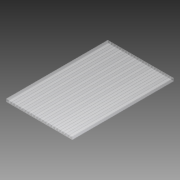
# Autodesk Inventor part: 8 ball polycarb side
Saved by Autodesk Inventor 2012 (Build 160160000, 160)
## iProperties
Created: 2013-10-11
Part Number: 8 ball polycarb side
Material: Default
Document SubType Name: Modeling
Designer: Bryce
Density: 1 g/cm^3
Author: Bryce
Autodesk Inventor part; units mm, degrees
ref_plane "YZ Plane" through (0, 0, 0) normal (1, 0, 0) x (0, 1, 0)
ref_plane "XZ Plane" through (0, 0, 0) normal (0, 1, 0) x (-1, 0, 0)
ref_plane "XY Plane" through (0, 0, 0) normal (0, 0, 1) x (1, 0, 0)
sketch "Sketch1" plane through (0, 0, 0) normal (0, 0, 1) x (1, 0, 0)
  line L0 (0, 0) -> (146.558, 0)
  line L1 (146.558, 0) -> (146.558, 6.35)
  line L2 (146.558, 6.35) -> (0, 6.35)
  line L3 (0, 6.35) -> (0, 0)
  line L4 (0.508, 0.5094) -> (6.35, 0.5094)
  line L5 (6.35, 0.5094) -> (6.35, 5.842)
  line L6 (6.35, 5.842) -> (0.508, 5.842)
  line L7 (0.508, 5.842) -> (0.508, 0.5094)
  line L8 (6.858, 0.5094) -> (12.7, 0.5094)
  line L9 (12.7, 0.5094) -> (12.7, 5.842)
  line L10 (12.7, 5.842) -> (6.858, 5.842)
  line L11 (6.858, 5.842) -> (6.858, 0.5094)
  line L12 (13.208, 0.5094) -> (19.05, 0.5094)
  line L13 (19.05, 0.5094) -> (19.05, 5.842)
  line L14 (19.05, 5.842) -> (13.208, 5.842)
  line L15 (13.208, 5.842) -> (13.208, 0.5094)
  line L16 (19.558, 0.5094) -> (25.4, 0.5094)
  line L17 (25.4, 0.5094) -> (25.4, 5.842)
  line L18 (25.4, 5.842) -> (19.558, 5.842)
  line L19 (19.558, 5.842) -> (19.558, 0.5094)
  line L20 (25.908, 0.5094) -> (31.75, 0.5094)
  line L21 (31.75, 0.5094) -> (31.75, 5.842)
  line L22 (31.75, 5.842) -> (25.908, 5.842)
  line L23 (25.908, 5.842) -> (25.908, 0.5094)
  line L24 (32.258, 0.5094) -> (38.1, 0.5094)
  line L25 (38.1, 0.5094) -> (38.1, 5.842)
  line L26 (38.1, 5.842) -> (32.258, 5.842)
  line L27 (32.258, 5.842) -> (32.258, 0.5094)
  line L28 (38.608, 0.5094) -> (44.45, 0.5094)
  line L29 (44.45, 0.5094) -> (44.45, 5.842)
  line L30 (44.45, 5.842) -> (38.608, 5.842)
  line L31 (38.608, 5.842) -> (38.608, 0.5094)
  line L32 (44.958, 0.5094) -> (50.8, 0.5094)
  line L33 (50.8, 0.5094) -> (50.8, 5.842)
  line L34 (50.8, 5.842) -> (44.958, 5.842)
  line L35 (44.958, 5.842) -> (44.958, 0.5094)
  line L36 (51.308, 0.5094) -> (57.15, 0.5094)
  line L37 (57.15, 0.5094) -> (57.15, 5.842)
  line L38 (57.15, 5.842) -> (51.308, 5.842)
  line L39 (51.308, 5.842) -> (51.308, 0.5094)
  line L40 (57.658, 0.5094) -> (63.5, 0.5094)
  line L41 (63.5, 0.5094) -> (63.5, 5.842)
  line L42 (63.5, 5.842) -> (57.658, 5.842)
  line L43 (57.658, 5.842) -> (57.658, 0.5094)
  line L44 (64.008, 0.5094) -> (69.85, 0.5094)
  line L45 (69.85, 0.5094) -> (69.85, 5.842)
  line L46 (69.85, 5.842) -> (64.008, 5.842)
  line L47 (64.008, 5.842) -> (64.008, 0.5094)
  line L48 (70.358, 0.5094) -> (76.2, 0.5094)
  line L49 (76.2, 0.5094) -> (76.2, 5.842)
  line L50 (76.2, 5.842) -> (70.358, 5.842)
  line L51 (70.358, 5.842) -> (70.358, 0.5094)
  line L52 (76.708, 0.5094) -> (82.55, 0.5094)
  line L53 (82.55, 0.5094) -> (82.55, 5.842)
  line L54 (82.55, 5.842) -> (76.708, 5.842)
  line L55 (76.708, 5.842) -> (76.708, 0.5094)
  line L56 (83.058, 0.5094) -> (88.9, 0.5094)
  line L57 (88.9, 0.5094) -> (88.9, 5.842)
  line L58 (88.9, 5.842) -> (83.058, 5.842)
  line L59 (83.058, 5.842) -> (83.058, 0.5094)
  line L60 (89.408, 0.5094) -> (95.25, 0.5094)
  line L61 (95.25, 0.5094) -> (95.25, 5.842)
  line L62 (95.25, 5.842) -> (89.408, 5.842)
  line L63 (89.408, 5.842) -> (89.408, 0.5094)
  line L64 (95.758, 0.5094) -> (101.6, 0.5094)
  line L65 (101.6, 0.5094) -> (101.6, 5.842)
  line L66 (101.6, 5.842) -> (95.758, 5.842)
  line L67 (95.758, 5.842) -> (95.758, 0.5094)
  line L68 (102.108, 0.5094) -> (107.95, 0.5094)
  line L69 (107.95, 0.5094) -> (107.95, 5.842)
  line L70 (107.95, 5.842) -> (102.108, 5.842)
  line L71 (102.108, 5.842) -> (102.108, 0.5094)
  line L72 (108.458, 0.5094) -> (114.3, 0.5094)
  line L73 (114.3, 0.5094) -> (114.3, 5.842)
  line L74 (114.3, 5.842) -> (108.458, 5.842)
  line L75 (108.458, 5.842) -> (108.458, 0.5094)
  line L76 (114.808, 0.5094) -> (120.65, 0.5094)
  line L77 (120.65, 0.5094) -> (120.65, 5.842)
  line L78 (120.65, 5.842) -> (114.808, 5.842)
  line L79 (114.808, 5.842) -> (114.808, 0.5094)
  line L80 (121.158, 0.5094) -> (127, 0.5094)
  line L81 (127, 0.5094) -> (127, 5.842)
  line L82 (127, 5.842) -> (121.158, 5.842)
  line L83 (121.158, 5.842) -> (121.158, 0.5094)
  line L84 (127.508, 0.5094) -> (133.35, 0.5094)
  line L85 (133.35, 0.5094) -> (133.35, 5.842)
  line L86 (133.35, 5.842) -> (127.508, 5.842)
  line L87 (127.508, 5.842) -> (127.508, 0.5094)
  line L88 (133.858, 0.5094) -> (139.7, 0.5094)
  line L89 (139.7, 0.5094) -> (139.7, 5.842)
  line L90 (139.7, 5.842) -> (133.858, 5.842)
  line L91 (133.858, 5.842) -> (133.858, 0.5094)
  line L92 (140.208, 0.5094) -> (146.05, 0.5094)
  line L93 (146.05, 0.5094) -> (146.05, 5.842)
  line L94 (146.05, 5.842) -> (140.208, 5.842)
  line L95 (140.208, 5.842) -> (140.208, 0.5094)
  dimension "d0" = 146.558
  dimension "d1" = 6.35
  dimension "d2" = 0.5094
  dimension "d3" = 0.508
  dimension "d4" = 0.508
  dimension "d5" = 5.842
  dimension "d8" = 6.35
  constraints: 192 end point, 4 parallel, 3 horizontal, 2 perpendicular, 176 other
  measures "d0" distance of L0.start L0.end
  measures "d1" distance of L2.end L0.start
  measures "d2" distance between parallel lines of L0 L4
  measures "d3" distance between parallel lines of L3 L7
  measures "d4" distance between parallel lines of L2 L6
  measures "d5" distance of L5.end L6.end
  measures "d8" distance of L5.end L10.start
extrude "Extrusion1" add sketch "Sketch1" along normal blind 225.425
body "Solid1"
